# Autodesk Inventor part: MCP3208-XX_SL
Saved by Autodesk Inventor 2013 (Build 170138000, 138)
## iProperties
Created: 2013-01-27
Part Number: MCP3208-XX_SL
Material: Generic
Document SubType Name: Modeling
Designer: davidgitz
Density: 1 g/cm^3
Author: davidgitz
Autodesk Inventor part; units mm, degrees
ref_plane "YZ Plane" through (0, 0, 0) normal (1, 0, 0) x (0, 1, 0)
ref_plane "XZ Plane" through (0, 0, 0) normal (0, 1, 0) x (-1, 0, 0)
ref_plane "XY Plane" through (0, 0, 0) normal (0, 0, 1) x (1, 0, 0)
sketch "SOIC16-N_MC, MCP3208-XX_SL_1" plane through (0, 0, 0) normal (0, 0, 1) x (1, 0, 0)
  line L0 (-3.3528, -5.0292) -> (3.3528, -5.0292)
  line L1 (3.3528, -5.0292) -> (3.3528, 5.0292)
  line L2 (3.3528, 5.0292) -> (-3.3528, 5.0292)
  line L3 (-3.3528, 5.0292) -> (-3.3528, -5.0292)
  constraints: 8 end point
extrude "Extrusion1" add sketch "SOIC16-N_MC, MCP3208-XX_SL_1" along normal blind 1
body "Solid1"
